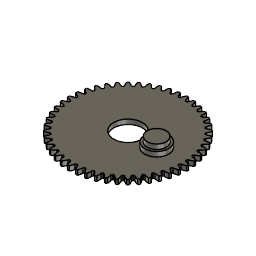
DriveGear (Autodesk Fusion 360 design; units mm, degrees)
description: Spur Gear; Module: 1.25; Num Teeth: 24; Pressure Angle: 20.0; Backlash: 0.00 mm
part number: 2026-05-31-22-10-19-992
Autodesk Fusion 360 part; units mm, degrees
sketch "Base Circle (1)" plane through (0, 0, 0) normal (0, 0, 1) x (1, 0, 0)
  circle A0 centre (0, 0) radius 11.4215
  circle A1 centre (0, 0) radius 3
  line L0 (0, 0) -> (6, 0)
  circle A2 centre (6, 0) radius 2
  circle A3 centre (6, 0) radius 2.5
  dimension "d27" = 6
  dimension "d30" = 4
  dimension "d31" = 6
  dimension "d34" = 5
  constraint coincident A0.centre A1.centre
  constraint horizontal L0
  constraint coincident L0.end A2.centre
  constraint concentric A2 A3
  measures "d27" diameter of A1
  measures "d30" diameter of A2
  measures "d31" distance of A0.centre L0.end
  measures "d34" diameter of A3
extrude "Extrude5" add sketch "Base Circle (1)" along normal blind 10 contours A0 | A2 | A3
sketch "Gear Tooth (1)" plane through (0, 0, 0) normal (0, 0, 1) x (1, 0, 0)
  spline S0 degree 5 poles (11.2635, -0.5369) (11.2671, -0.5369) (11.2741, -0.5369) (11.2847, -0.5368) (11.2989, -0.5365) (11.3166, -0.5359) (11.3343, -0.535) (11.352, -0.5338) (11.3697, -0.5323) (11.3874, -0.5306) (11.4051, -0.5287) (11.4228, -0.5266) (11.4406, -0.5244) (11.4583, -0.522) (11.476, -0.5194) (11.4937, -0.5167) (11.5115, -0.5139) (11.5292, -0.5109) (11.5469, -0.5078) (11.5647, -0.5046) (11.5824, -0.5012) (11.6001, -0.4977) (11.6178, -0.4941) (11.6356, -0.4904) (11.6533, -0.4865) (11.671, -0.4826) (11.6887, -0.4785) (11.7064, -0.4743) (11.7241, -0.47) (11.7418, -0.4657) (11.7596, -0.4612) (11.7773, -0.4566) (11.795, -0.4519) (11.8127, -0.4471) (11.8303, -0.4422) (11.848, -0.4372) (11.8657, -0.4321) (11.8834, -0.427) (11.9011, -0.4217) (11.9188, -0.4163) (11.9364, -0.4109) (11.9541, -0.4054) (11.9717, -0.3997) (11.9894, -0.394) (12.007, -0.3882) (12.0247, -0.3823) (12.0423, -0.3764) (12.06, -0.3703) (12.0776, -0.3642) (12.0952, -0.3579) (12.1128, -0.3516) (12.1304, -0.3452) (12.148, -0.3388) (12.1656, -0.3322) (12.1832, -0.3256) (12.2008, -0.3189) (12.2184, -0.3121) (12.2359, -0.3052) (12.2535, -0.2983) (12.271, -0.2913) (12.2886, -0.2842) (12.3061, -0.277) (12.3237, -0.2698) (12.3412, -0.2625) (12.3587, -0.2551) (12.3762, -0.2476) (12.3937, -0.24) (12.4112, -0.2324) (12.4287, -0.2247) (12.4461, -0.217) (12.4636, -0.2091) (12.4776, -0.2028) (12.488, -0.198) (12.495, -0.1948) (12.4985, -0.1932) knots 0 0 0 0 0 0 0.01428571 0.02857143 0.04285714 0.05714286 0.07142857 0.08571429 0.1 0.11428571 0.12857143 0.14285714 0.15714286 0.17142857 0.18571429 0.2 0.21428571 0.22857143 0.24285714 0.25714286 0.27142857 0.28571429 0.3 0.31428571 0.32857143 0.34285714 0.35714286 0.37142857 0.38571429 0.4 0.41428571 0.42857143 0.44285714 0.45714286 0.47142857 0.48571429 0.5 0.51428571 0.52857143 0.54285714 0.55714286 0.57142857 0.58571429 0.6 0.61428571 0.62857143 0.64285714 0.65714286 0.67142857 0.68571429 0.7 0.71428571 0.72857143 0.74285714 0.75714286 0.77142857 0.78571429 0.8 0.81428571 0.82857143 0.84285714 0.85714286 0.87142857 0.88571429 0.9 0.91428571 0.92857143 0.94285714 0.95714286 0.97142857 0.98571429 1 1 1 1 1 1
  spline S1 degree 5 poles (11.2635, 0.5369) (11.2671, 0.5369) (11.2741, 0.5369) (11.2847, 0.5368) (11.2989, 0.5365) (11.3166, 0.5359) (11.3343, 0.535) (11.352, 0.5338) (11.3697, 0.5323) (11.3874, 0.5306) (11.4051, 0.5287) (11.4228, 0.5266) (11.4406, 0.5244) (11.4583, 0.522) (11.476, 0.5194) (11.4937, 0.5167) (11.5115, 0.5139) (11.5292, 0.5109) (11.5469, 0.5078) (11.5647, 0.5046) (11.5824, 0.5012) (11.6001, 0.4977) (11.6178, 0.4941) (11.6356, 0.4904) (11.6533, 0.4865) (11.671, 0.4826) (11.6887, 0.4785) (11.7064, 0.4743) (11.7241, 0.47) (11.7418, 0.4657) (11.7596, 0.4612) (11.7773, 0.4566) (11.795, 0.4519) (11.8127, 0.4471) (11.8303, 0.4422) (11.848, 0.4372) (11.8657, 0.4321) (11.8834, 0.427) (11.9011, 0.4217) (11.9188, 0.4163) (11.9364, 0.4109) (11.9541, 0.4054) (11.9717, 0.3997) (11.9894, 0.394) (12.007, 0.3882) (12.0247, 0.3823) (12.0423, 0.3764) (12.06, 0.3703) (12.0776, 0.3642) (12.0952, 0.3579) (12.1128, 0.3516) (12.1304, 0.3452) (12.148, 0.3388) (12.1656, 0.3322) (12.1832, 0.3256) (12.2008, 0.3189) (12.2184, 0.3121) (12.2359, 0.3052) (12.2535, 0.2983) (12.271, 0.2913) (12.2886, 0.2842) (12.3061, 0.277) (12.3237, 0.2698) (12.3412, 0.2625) (12.3587, 0.2551) (12.3762, 0.2476) (12.3937, 0.24) (12.4112, 0.2324) (12.4287, 0.2247) (12.4461, 0.217) (12.4636, 0.2091) (12.4776, 0.2028) (12.488, 0.198) (12.495, 0.1948) (12.4985, 0.1932) knots 0 0 0 0 0 0 0.01428571 0.02857143 0.04285714 0.05714286 0.07142857 0.08571429 0.1 0.11428571 0.12857143 0.14285714 0.15714286 0.17142857 0.18571429 0.2 0.21428571 0.22857143 0.24285714 0.25714286 0.27142857 0.28571429 0.3 0.31428571 0.32857143 0.34285714 0.35714286 0.37142857 0.38571429 0.4 0.41428571 0.42857143 0.44285714 0.45714286 0.47142857 0.48571429 0.5 0.51428571 0.52857143 0.54285714 0.55714286 0.57142857 0.58571429 0.6 0.61428571 0.62857143 0.64285714 0.65714286 0.67142857 0.68571429 0.7 0.71428571 0.72857143 0.74285714 0.75714286 0.77142857 0.78571429 0.8 0.81428571 0.82857143 0.84285714 0.85714286 0.87142857 0.88571429 0.9 0.91428571 0.92857143 0.94285714 0.95714286 0.97142857 0.98571429 1 1 1 1 1 1
  arc A0 (12.4985, -0.1932) -> (12.4985, 0.1932) centre (0, 0) ccw
  line L0 (11.2635, 0.5369) -> (11.2635, -0.5369)
  point P0 (11.3512, -0.5338)
  point P1 (11.4391, -0.5245)
  point P2 (11.5272, -0.5112)
  point P3 (11.6154, -0.4946)
  point P4 (11.7037, -0.4749)
  point P5 (11.7921, -0.4526)
  point P6 (11.8805, -0.4278)
  point P7 (11.9689, -0.4006)
  point P8 (12.0573, -0.3712)
  point P9 (12.1456, -0.3396)
  point P10 (12.234, -0.306)
  point P11 (12.3222, -0.2703)
  point P12 (12.4104, -0.2327)
  point P13 (11.3512, 0.5338)
  point P14 (11.4391, 0.5245)
  point P15 (11.5272, 0.5112)
  point P16 (11.6154, 0.4946)
  point P17 (11.7037, 0.4749)
  point P18 (11.7921, 0.4526)
  point P19 (11.8805, 0.4278)
  point P20 (11.9689, 0.4006)
  point P21 (12.0573, 0.3712)
  point P22 (12.1456, 0.3396)
  point P23 (12.234, 0.306)
  point P24 (12.3222, 0.2703)
  point P25 (12.4104, 0.2327)
extrude "Extrude6" add sketch "Gear Tooth (1)" along normal blind 10
fillet "Fillet3" radius 0.25 2 edges at (11.4093, 0.5282, 5) (11.4093, -0.5282, 5)
pattern_circular "C-Pattern3" count 48 over 360 about axis through (0, 0, 0) along (0, 0, 1) of "Extrude6", "Fillet3"
sketch "Diametrial Pitch Circle (1)" plane through (0, 0, 0) normal (0, 0, 1) x (1, 0, 0)
  circle A0 centre (0, 0) radius 12 construction
extrude "Extrude7" cut 1 faces at (-4.2994, -7.4469, 10) along direction (0, 0, -1) blind 9
extrude "Extrude8" add sketch "Base Circle (1)" along normal blind 3 contours A2
extrude "Extrude9" add sketch "Base Circle (1)" along normal blind 2 contours A2 | A3
named bodies: "Spur Gear (48 teeth)"
